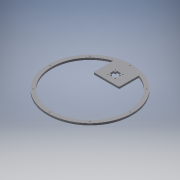
# Autodesk Inventor part: Base_Acryllic
Saved by Autodesk Inventor 2016 (Build 200138000, 138)
## iProperties
Created: 2016-03-29
Part Number: Base_Acryllic
Material: Generic
Document SubType Name: Modeling
Designer: Ethan
Density: 1 g/cm^3
Appearance: Default
Author: Ethan
Autodesk Inventor part; units mm, degrees
ref_plane "YZ Plane" through (0, 0, 0) normal (1, 0, 0) x (0, 1, 0)
ref_plane "XZ Plane" through (0, 0, 0) normal (0, 1, 0) x (-1, 0, 0)
ref_plane "XY Plane" through (0, 0, 0) normal (0, 0, 1) x (1, 0, 0)
sketch "Sketch1" plane through (0, 0, 0) normal (0, 1, 0) x (-1, 0, 0)
  arc A0 (42.6787, -133.0211) -> (-42.6787, -133.0211) centre (0, 0) ccw
  circle A1 centre (2.7003, 146.7014) radius 1.5875
  line L0 (0, -97.1997) -> (0, -97.2112)
  circle A2 centre (0, -133.35) radius 1.5875
  circle A3 centre (94.2927, -94.2927) radius 1.5875
  circle A4 centre (133.35, 0) radius 1.5875
  circle A5 centre (94.2927, 94.2927) radius 1.5875
  circle A6 centre (0, 133.35) radius 1.5875
  circle A7 centre (-94.2927, 94.2927) radius 1.5875
  circle A8 centre (-133.35, 0) radius 1.5875
  circle A9 centre (-94.2927, -94.2927) radius 1.5875
  arc A10 (42.6787, -119.6141) -> (-42.8213, -119.5631) centre (0, 0) ccw
  line L1 (1.5875, -133.35) -> (-1.5875, -133.35)
  circle A11 centre (-12.5713, -96.7482) radius 1.5875
  circle A12 centre (12.4287, -96.7482) radius 1.5875
  circle A13 centre (-12.5713, -71.7482) radius 1.5875
  circle A14 centre (12.4287, -71.7482) radius 1.5875
  line L2 (-42.8213, -119.5631) -> (-42.8213, -57.4232)
  line L3 (-39.6463, -54.2482) -> (39.5037, -54.2482)
  line L4 (-12.5713, -77.8982) -> (-12.5713, -90.5982)
  line L5 (-6.4213, -96.7482) -> (6.2787, -96.7482)
  line L6 (6.2787, -71.7482) -> (-6.4213, -71.7482)
  line L7 (12.4167, -90.5982) -> (12.4167, -77.8982)
  line L8 (6.2787, -96.7482) -> (6.2787, -90.5982)
  line L9 (6.2787, -77.8982) -> (6.2787, -71.7482)
  line L10 (12.4167, -77.8982) -> (6.2787, -77.8982)
  line L11 (-6.4213, -77.8982) -> (-12.5713, -77.8982)
  line L12 (-6.4213, -71.7482) -> (-6.4213, -77.8982)
  line L13 (-6.4213, -90.5982) -> (-6.4213, -96.7482)
  line L14 (-12.5713, -90.5982) -> (-6.4213, -90.5982)
  line L15 (6.2787, -90.5982) -> (12.4167, -90.5982)
  line L16 (6.2787, -71.7482) -> (-6.4213, -71.7482)
  line L17 (-6.4213, -71.7482) -> (-6.4213, -96.7482)
  line L18 (-6.4213, -96.7482) -> (6.2787, -96.7482)
  line L19 (6.2787, -96.7482) -> (6.2787, -71.7482)
  line L20 (12.4167, -77.8982) -> (-12.5713, -77.8982)
  line L21 (-12.5713, -77.8982) -> (-12.5713, -90.5982)
  line L22 (-12.5713, -90.5982) -> (12.4167, -90.5982)
  line L23 (12.4167, -90.5982) -> (12.4167, -77.8982)
  line L24 (42.6787, -57.4232) -> (42.6787, -119.6141)
  arc A15 (-42.8213, -132.9753) -> (42.6787, -133.0211) centre (0, 0) ccw
  arc A16 (-39.6463, -54.2482) -> (-42.8213, -57.4232) centre (-39.6463, -57.4232) ccw
  arc A17 (42.6787, -57.4232) -> (39.5037, -54.2482) centre (39.5037, -57.4232) ccw
  point P0 (-42.8213, -54.2482)
  point P1 (42.6787, -54.2482)
  dimension "d0" = 279.4
  dimension "d97" = 3.175
  dimension "d134" = 3.175
  dimension "d135" = 133.35
  dimension "d138" = 360
  dimension "d140" = 254
  dimension "d156" = 3.175
  constraints: 50 end point, 18 centre point, 13 point on circle, 4 point on line, 4 tangent, 2 coincident, 1 equal radius, 1 horizontal, 17 other
  measures "d0" diameter of A0
  measures "d97" diameter of A1
  measures "d134" diameter of A2
  measures "d135" distance of point (0, 0) A2.centre
  measures "d140" diameter of A10
  measures "d156" radius of A16
extrude "Extrusion12" add sketch "Sketch1" along normal blind 6.35 contours A15 A0
body "Solid10"
